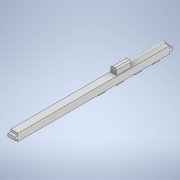
# Autodesk Inventor part: центр пушки
Saved by Autodesk Inventor 2020.1 (Build 241239000, 239)
## iProperties
Created: 2022-03-19
Part Number: центр пушки
Material: Типовые
Document SubType Name: Modeling
Designer: User
Density: 1 g/cm^3
Appearance: По умолчанию
Author: User
Autodesk Inventor part; units mm, degrees
ref_plane "YZ Plane" through (0, 0, 0) normal (1, 0, 0) x (0, 1, 0)
ref_plane "XZ Plane" through (0, 0, 0) normal (0, 1, 0) x (-1, 0, 0)
ref_plane "XY Plane" through (0, 0, 0) normal (0, 0, 1) x (1, 0, 0)
sketch "Эскиз1" plane through (0, 0, 0) normal (0, 0, 1) x (1, 0, 0)
  line L0 (0, 0) -> (-10, 0)
  line L1 (-10, 0) -> (-10, 10)
  line L2 (-10, 10) -> (0, 10)
  line L3 (0, 10) -> (0, 0)
  dimension "d0" = 10
  dimension "d1" = 10
  constraints: 8 end point, 2 parallel, 1 horizontal, 1 perpendicular
  measures "d0" distance of L1.end L2.end
  measures "d1" distance of L0.end L1.end
extrude "Выдавливание1" add sketch "Эскиз1" along normal blind 210
sketch "Эскиз2" plane through (0, 0, 210) normal (0, 0, 1) x (1, 0, 0)
  line L0 (-10, 10) -> (-10, 0) projected
  line L1 (0, 0) -> (0, 10) projected
  line L2 (-10, 3) -> (0, 3)
  line L3 (0, 3) -> (0, 7)
  line L4 (0, 7) -> (-10, 7)
  line L5 (-10, 7) -> (-10, 3)
  line L6 (-10, 5) -> (0, 5)
  point P0 (0, 3)
  dimension "d4" = 4
  constraints: 10 end point, 2 midpoint, 2 parallel, 2 point on line, 1 horizontal, 1 perpendicular, 1 other
  measures "d4" distance of L2.end L3.end
extrude "Выдавливание2" add sketch "Эскиз2" along normal blind 4
sketch "Эскиз3" plane through (0, 0, 0) normal (0, 0, -1) x (-1, 0, 0)
  line L0 (10, 7) -> (10, 3) projected
  line L1 (0, 0) -> (0, 3) projected
  line L2 (10, 7) -> (0, 7)
  line L3 (0, 7) -> (0, 3)
  line L4 (0, 3) -> (10, 3)
  line L5 (10, 3) -> (10, 7)
  constraints: 8 end point, 2 parallel, 1 horizontal, 1 perpendicular
extrude "Выдавливание3" add sketch "Эскиз3" along normal blind 4
sketch "Эскиз4" plane through (-10, 0, 0) normal (0, -1, 0) x (1, 0, 0)
  line L0 (10, 0) -> (10, 210) projected
  line L1 (10, 105) -> (0, 105)
  line L2 (0, 0) -> (0, 210) projected
  line L3 (5, 105) -> (5, 0)
  line L4 (0, 0) -> (10, 0) projected
  line L5 (6.7537, 95) -> (3.2463, 95)
  line L6 (3.2463, 95) -> (3.2463, 85)
  line L7 (3.2463, 85) -> (6.7537, 85)
  line L8 (6.7537, 85) -> (6.7537, 95)
  line L9 (7.0866, 70) -> (2.9134, 70)
  line L10 (2.9134, 70) -> (2.9134, 60)
  line L11 (2.9134, 60) -> (7.0866, 60)
  line L12 (7.0866, 60) -> (7.0866, 70)
  line L13 (7.0866, 45) -> (2.9134, 45)
  line L14 (2.9134, 45) -> (2.9134, 35)
  line L15 (2.9134, 35) -> (7.0866, 35)
  line L16 (7.0866, 35) -> (7.0866, 45)
  line L17 (6.7537, 20) -> (3.2463, 20)
  line L18 (3.2463, 20) -> (3.2463, 10)
  line L19 (3.2463, 10) -> (6.7537, 10)
  line L20 (6.7537, 10) -> (6.7537, 20)
  dimension "d9" = 10
  dimension "d10" = 10
  dimension "d11" = 10
  dimension "d12" = 10
  dimension "d13" = 10
  dimension "d14" = 15
  dimension "d15" = 15
  dimension "d16" = 15
  constraints: 36 end point, 8 parallel, 4 horizontal, 4 midpoint, 4 perpendicular, 2 point on line, 4 other
  measures "d9" distance of L7.end L5.start
  measures "d10" distance of L11.end L9.start
  measures "d11" distance of L15.end L13.start
  measures "d12" distance of L19.end L17.start
  measures "d13" distance from line of L1 L5.start
  measures "d14" vertical distance of L9.start L7.end
  measures "d15" distance of L13.start L11.end
  measures "d16" vertical distance of L17.start L15.end
extrude "Выдавливание4" add sketch "Эскиз4" along normal blind 4 contours L19 L18 L17 L3 | L3 L17 L20 L19 | L5 L8 L7 L3 | L3 L7 L6 L5 | L15 L14 L13 L3 | L3 L13 L16 L15 | L9 L12 L11 L3 | L3 L11 L10 L9
sketch "Эскиз5" plane through (-10, 10, 0) normal (0, 1, 0) x (1, 0, 0)
  line L0 (9, -52.1164) -> (1, -52.1164)
  line L1 (1, -52.1164) -> (1, -72.1164)
  line L2 (1, -72.1164) -> (9, -72.1164)
  line L3 (9, -72.1164) -> (9, -52.1164)
  point P0 (10, 0)
  point P1 (10, -52.1164)
  dimension "d19" = 8
  dimension "d20" = 20
  dimension "d21" = 1
  constraints: 8 end point, 2 parallel, 1 horizontal, 1 perpendicular, 1 other
  measures "d19" distance of L0.start L0.end
  measures "d20" distance of L0.end L1.end
  measures "d21" distance of point (10, -52.116) L0.start
extrude "Выдавливание5" add sketch "Эскиз5" along normal blind 8
fillet "Сопряжение1" radius 2 2 edges at (-1, 18, 62.1164) (-9, 18, 62.1164)
sketch "Эскиз6" plane through (-1, 10, 52.1164) normal (0, 0, -1) x (-1, 0, 0)
  line L0 (2, 8) -> (6, 8) projected
  line L1 (8, 0) -> (8, 6) projected
  circle A0 centre (4, 3) radius 1.5
  point P0 (-1, -10)
  point P1 (4, 8)
  point P2 (8, 3)
  dimension "d25" = 3
  constraints: 2 midpoint, 1 centre point
  measures "d25" diameter of A0
extrude "Выдавливание6" add sketch "Эскиз6" along normal blind 50
